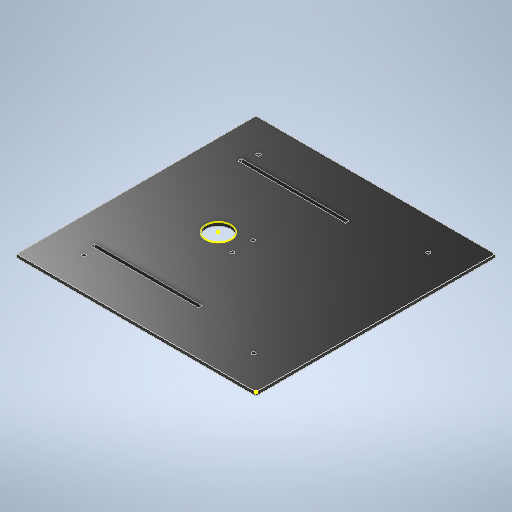
# Autodesk Inventor part: Part 1 base
Saved by Autodesk Inventor 2025.4 (Build 294407000, 407)
## iProperties
Created: 2026-04-06
Part Number: Part 1 base
Material: Generic
Document SubType Name: Modeling
Designer: abdo2
Density: 1 g/cm^3
Appearance: Glossy - Black
Author: abdo2
Autodesk Inventor part; units mm, degrees
ref_plane "YZ Plane" through (0, 0, 0) normal (1, 0, 0) x (0, 1, 0)
ref_plane "XZ Plane" through (0, 0, 0) normal (0, 1, 0) x (-1, 0, 0)
ref_plane "XY Plane" through (0, 0, 0) normal (0, 0, 1) x (1, 0, 0)
sketch "Sketch1" plane through (0, 0, 0) normal (0, 1, 0) x (-1, 0, 0)
  line L0 (0, 0) -> (200, 0)
  line L1 (200, 0) -> (200, -200)
  line L2 (200, -200) -> (0, -200)
  line L3 (0, -200) -> (0, 0)
  dimension "d0" = 200
  dimension "d1" = 200
  constraints: 8 end point, 2 parallel, 1 horizontal, 1 perpendicular
  measures "d0" distance of L1.end L2.end
  measures "d1" distance of L0.end L1.end
extrude "Extrusion1" add sketch "Sketch1" along normal blind 3
sketch "Sketch4" plane through (0, 3, 0) normal (0, 1, 0) x (1, 0, 0)
  line L0 (-175, 37) -> (-175, 40)
  line L1 (-175, 40) -> (-85, 40)
  line L2 (-85, 40) -> (-85, 37)
  line L3 (-85, 37) -> (-175, 37)
  line L4 (-190, 6) -> (-10, 6) projected
  line L5 (-200, 200) -> (-200, 0) projected
  line L6 (-175, 160) -> (-175, 163)
  line L7 (-175, 163) -> (-85, 163)
  line L8 (-85, 163) -> (-85, 160)
  line L9 (-85, 160) -> (-175, 160)
  line L10 (0, 0) -> (0, 200) projected
  line L11 (-10, 194) -> (-190, 194) projected
  dimension "d24" = 3
  dimension "d25" = 90
  dimension "d26" = 31
  dimension "d27" = 25
  dimension "d28" = 3
  dimension "d29" = 120
  dimension "d30" = 25
  dimension "d31" = 85
  dimension "d52" = 31
  constraints: 16 end point, 5 perpendicular, 2 vertical, 1 parallel
  measures "d24" distance of L0.start L0.end
  measures "d25" distance of L0.end L1.end
  measures "d26" distance between parallel lines of L4 L3
  measures "d27" distance between parallel lines of L5 L0
  measures "d28" distance of L6.start L6.end
  measures "d29" distance between parallel lines of L9 L1
  measures "d30" distance between parallel lines of L5 L6
  measures "d31" distance between parallel lines of L10 L8
  measures "d52" distance from line of L11 L7.end
extrude "Extrusion4" cut sketch "Sketch4" against normal blind 3
sketch "Sketch5" plane through (0, 3, 0) normal (0, 1, 0) x (1, 0, 0)
  circle A0 centre (-131.5, 100) radius 10.5
  line L0 (-200, 200) -> (-200, 0) projected
  line L1 (-175, 40) -> (-85, 40) projected
  line L2 (-175, 160) -> (-175, 163) projected
  line L3 (-85, 160) -> (-175, 160) projected
  point P0 (0, 0)
  dimension "d34" = 21
  dimension "d37" = 60
  dimension "d40" = 43.5
  dimension "d53" = 60
  constraints: 1 centre point
  measures "d34" diameter of A0
  measures "d37" distance from line of L1 A0.centre
  measures "d40" distance from line of L2 A0.centre
  measures "d53" distance from line of A0.centre L3
extrude "Extrusion5" cut sketch "Sketch5" against normal blind 10
sketch "Sketch8" plane through (0, 3, 0) normal (0, 1, 0) x (1, 0, 0)
  circle A0 centre (-131.5, 100) radius 10.5 projected
  point P0 (0, 0)
sketch "Sketch11" plane through (0, 3, 0) normal (0, 1, 0) x (1, 0, 0)
  line L0 (-111, 108.75) -> (-111, 91.25)
  circle A0 centre (-131.5, 100) radius 10.5 projected
  circle A1 centre (-111, 108.75) radius 1.5
  circle A2 centre (-111, 91.25) radius 1.5
  point P0 (0, 0)
  dimension "d60" = 20.5
  dimension "d61" = 3
  dimension "d62" = 3
  dimension "d63" = 17.5
  dimension "d64" = 8.75
  constraints: 2 centre point, 2 coincident, 2 end point, 1 vertical
  measures "d60" distance from line of A0.centre L0
  measures "d61" diameter of A1
  measures "d62" diameter of A2
  measures "d63" distance of L0.end L0.start
  measures "d64" vertical distance of L0.end A0.centre
extrude "Extrusion8" cut sketch "Sketch11" against normal blind 10 contours A2 | A1
sketch "Sketch12" plane through (0, 3, 0) normal (0, 1, 0) x (1, 0, 0)
  circle A0 centre (-171, 27) radius 1.6
  line L0 (-194, 190) -> (-194, 10) projected
  line L1 (-190, 6) -> (-10, 6) projected
  circle A1 centre (-171, 173) radius 1.6
  line L2 (-10, 194) -> (-190, 194) projected
  circle A2 centre (-29, 27) radius 1.6
  line L3 (-6, 10) -> (-6, 190) projected
  circle A3 centre (-29, 173) radius 1.6
  point P0 (0, 0)
  dimension "d67" = 3.2
  dimension "d68" = 23
  dimension "d69" = 21
  dimension "d70" = 3.2
  dimension "d71" = 21
  dimension "d72" = 23
  dimension "d73" = 3.2
  dimension "d74" = 21
  dimension "d75" = 23
  dimension "d76" = 3.2
  dimension "d77" = 21
  dimension "d78" = 23
  constraints: 4 centre point
  measures "d67" diameter of A0
  measures "d68" distance from line of L0 A0.centre
  measures "d69" distance from line of A0.centre L1
  measures "d70" diameter of A1
  measures "d71" distance from line of L2 A1.centre
  measures "d72" distance from line of L0 A1.centre
  measures "d73" diameter of A2
  measures "d74" distance from line of L1 A2.centre
  measures "d75" distance from line of L3 A2.centre
  measures "d76" diameter of A3
  measures "d77" distance from line of L2 A3.centre
  measures "d78" distance from line of L3 A3.centre
extrude "Extrusion9" cut sketch "Sketch12" against normal blind 10
equation "\"d26\" = d52"
equation "\"d37\" = d53"
body "Solid1"
